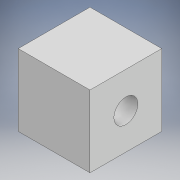
# Autodesk Inventor part: RaDecConnector
Saved by Autodesk Inventor 2022 (Build 260153000, 153)
## iProperties
Created: 2021-05-01
Part Number: RaDecConnector
Material: Generic
Document SubType Name: Modeling
Designer: Mick Veldhuis
Density: 1 g/cm^3
Appearance: Default
Author: Mick Veldhuis
Autodesk Inventor part; units mm, degrees
ref_plane "YZ Plane" through (0, 0, 0) normal (1, 0, 0) x (0, 1, 0)
ref_plane "XZ Plane" through (0, 0, 0) normal (0, 1, 0) x (-1, 0, 0)
ref_plane "XY Plane" through (0, 0, 0) normal (0, 0, 1) x (1, 0, 0)
sketch "Sketch1" plane through (0, 0, 0) normal (0, 1, 0) x (-1, 0, 0)
  line L0 (99, 99) -> (-99, 99)
  line L1 (-99, 99) -> (-99, -99)
  line L2 (-99, -99) -> (99, -99)
  line L3 (99, -99) -> (99, 99)
  line L4 (99, 99) -> (-99, -99) construction
  line L5 (-99, 99) -> (99, -99) construction
  point P0 (0, 0)
  dimension "d0" = 198
  dimension "d1" = 198
  constraints: 12 end point, 2 midpoint, 2 parallel, 1 horizontal, 1 perpendicular
  measures "d0" distance of L2.end L1.end
  measures "d1" distance of L1.end L0.end
extrude "Box" add sketch "Sketch1" along normal blind 198
sketch "Sketch2" plane through (99, 0, 99) normal (1, 0, 0) x (0, 0, -1)
  point P0 (99, 0)
  point P1 (99, 99)
hole "DecAxisHole" at (99, 99, 0) direction (-1, 0, 0) diameter 66 depth 198
sketch "Sketch3" plane through (0, 0, 0) normal (0, -1, 0) x (1, 0, 0)
  point P0 (0, 0)
  point P1 (-76, -76)
  point P2 (76, -76)
  point P3 (76, 76)
  point P4 (-76, 76)
hole "BoltHoles" at (-76, 0, -76) at (76, 0, -76) at (76, 0, 76) at (-76, 0, 76) direction (0, 1, 0) diameter 8 depth 24 tip angle 118
body "Solid1"
